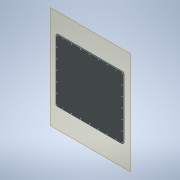
# Autodesk Inventor part: Крышка картера 2
Saved by Autodesk Inventor 2021 (Build 250183000, 183)
## iProperties
Created: 2020-12-12
Part Number: Крышка картера 2
Material: Чугун, серый
Document SubType Name: Modeling
Designer: Тимоха
Mass: 32984 g
Surface Area: 9566.62 cm^2
Volume: 4613.15 cm^3
Density: 7.15 g/cm^3
Appearance: Чугун серый
Author: Тимоха
Autodesk Inventor part; units mm, degrees
ref_plane "YZ Plane" through (0, 0, 0) normal (1, 0, 0) x (0, 1, 0)
ref_plane "XZ Plane" through (0, 0, 0) normal (0, 1, 0) x (-1, 0, 0)
ref_plane "XY Plane" through (0, 0, 0) normal (0, 0, 1) x (1, 0, 0)
ref_plane "РабПлоскость1" through (0, 0, 0) normal (0, 0, 1) x (1, 0, 0)
sketch "Эскиз1" plane through (0, 0, 0) normal (0, 0, 1) x (1, 0, 0)
  circle A0 centre (340, 472) radius 4 projected
  circle A1 centre (340, 367) radius 4 projected
  circle A2 centre (340, 322.8) radius 4 projected
  circle A3 centre (340, 218.5) radius 4 projected
  circle A4 centre (340, 114.2) radius 4 projected
  circle A5 centre (340, 9.9) radius 4 projected
  circle A6 centre (340, -94.4) radius 4 projected
  circle A7 centre (340, -198.7) radius 4 projected
  circle A8 centre (340, -303) radius 4 projected
  circle A9 centre (340, -347) radius 4 projected
  circle A10 centre (340, -407) radius 4 projected
  circle A11 centre (340, -467) radius 4 projected
  circle A12 centre (278, 472) radius 4 projected
  circle A13 centre (185, 472) radius 4 projected
  circle A14 centre (92, 472) radius 4 projected
  circle A15 centre (-1, 472) radius 4 projected
  circle A16 centre (-94, 472) radius 4 projected
  circle A17 centre (-187, 472) radius 4 projected
  circle A18 centre (-280, 472) radius 4 projected
  circle A19 centre (-340, 472) radius 4 projected
  circle A20 centre (-340, 367) radius 4 projected
  circle A21 centre (-340, 322.8) radius 4 projected
  circle A22 centre (-340, 218.5) radius 4 projected
  circle A23 centre (-340, 114.2) radius 4 projected
  circle A24 centre (-340, 9.9) radius 4 projected
  circle A25 centre (-340, -94.4) radius 4 projected
  circle A26 centre (-340, -198.7) radius 4 projected
  circle A27 centre (-340, -303) radius 4 projected
  circle A28 centre (-340, -347) radius 4 projected
  circle A29 centre (-340, -407) radius 4 projected
  circle A30 centre (-340, -467) radius 4 projected
  line L0 (165, -460) -> (165, -485) projected
  line L1 (185, -485) -> (165, -485) projected
  line L2 (185, -475) -> (185, -485) projected
  line L3 (185, -475) -> (380, -475) projected
  line L4 (380, -475) -> (380, 475) projected
  line L5 (380, 475) -> (350, 475) projected
  line L6 (350, 475) -> (350, 485) projected
  line L7 (-350, 485) -> (350, 485) projected
  line L8 (-350, 475) -> (-350, 485) projected
  line L9 (-350, 475) -> (-380, 475) projected
  line L10 (-380, 475) -> (-380, -475) projected
  line L11 (-380, -475) -> (-185, -475) projected
  line L12 (-185, -475) -> (-185, -485) projected
  line L13 (-165, -485) -> (-185, -485) projected
  line L14 (-165, -485) -> (-165, -460) projected
  line L15 (-165, -460) -> (-330, -460) projected
  line L16 (-330, 460) -> (-330, -460) projected
  line L17 (-330, 460) -> (330, 460) projected
  line L18 (330, -460) -> (330, 460) projected
  line L19 (330, -460) -> (165, -460) projected
  circle A31 centre (278, -303) radius 4 projected
  circle A32 centre (185, -303) radius 4 projected
  circle A33 centre (92, -303) radius 4 projected
  circle A34 centre (-1, -303) radius 4 projected
  circle A35 centre (-94, -303) radius 4 projected
  circle A36 centre (-187, -303) radius 4 projected
  circle A37 centre (-280, -303) radius 4 projected
  circle A38 centre (278, -347) radius 4 projected
  circle A39 centre (185, -347) radius 4 projected
  circle A40 centre (92, -347) radius 4 projected
  circle A41 centre (-1, -347) radius 4 projected
  circle A42 centre (-94, -347) radius 4 projected
  circle A43 centre (-187, -347) radius 4 projected
  circle A44 centre (-280, -347) radius 4 projected
  line L20 (-330, -291) -> (-330, -359) projected
  line L21 (-330, -359) -> (330, -359) projected
  line L22 (330, -291) -> (330, -359) projected
  line L23 (-330, -291) -> (330, -291) projected
  circle A45 centre (278, 367) radius 4 projected
  circle A46 centre (185, 367) radius 4 projected
  circle A47 centre (92, 367) radius 4 projected
  circle A48 centre (-1, 367) radius 4 projected
  circle A49 centre (-94, 367) radius 4 projected
  circle A50 centre (-187, 367) radius 4 projected
  circle A51 centre (-280, 367) radius 4 projected
  circle A52 centre (278, 323) radius 4 projected
  circle A53 centre (185, 323) radius 4 projected
  circle A54 centre (92, 323) radius 4 projected
  circle A55 centre (-1, 323) radius 4 projected
  circle A56 centre (-94, 323) radius 4 projected
  circle A57 centre (-187, 323) radius 4 projected
  circle A58 centre (-280, 323) radius 4 projected
  line L24 (-330, 379) -> (-330, 311) projected
  line L25 (-330, 311) -> (330, 311) projected
  line L26 (330, 379) -> (330, 311) projected
  line L27 (-330, 379) -> (330, 379) projected
  circle A59 centre (-340, 322.8) radius 14
  circle A60 centre (-340, -303) radius 14
  circle A61 centre (340, -303) radius 14
  circle A62 centre (340, 322.8) radius 14
  line L28 (340, 336.8) -> (-340, 336.8)
  line L29 (-354, 322.8) -> (-354, -303)
  line L30 (-340, -317) -> (340, -317)
  line L31 (354, -303) -> (354, 322.8)
  point P0 (0, 0)
  dimension "d0" = 10
  dimension "d1" = 10
  dimension "d2" = 10
  dimension "d3" = 10
  constraints: 8 end point, 8 point on circle, 5 tangent, 4 centre point
  measures "d0" radial gap between concentric circles of A21 A59
  measures "d1" radial gap between concentric circles of A27 A60
  measures "d2" radial gap between concentric circles of A8 A61
  measures "d3" radial gap between concentric circles of A2 A62
extrude "Выдавливание1" add sketch "Эскиз1" along normal blind 10 contours L30 L16 A60 L23 L18 A61 | L18 A61 L30 | A61 L18 | L18 A61 | L30 A60 L16 | L18 A62 L31 A61 | A60 L16 | L16 A60 | L23 L16 L25 L18 | A60 L29 A59 L16 | A62 L18 | L25 L16 A59 L28 L18 A62 | A59 L16 | A62 L18 L28 | A62 L18 | L28 L16 A59 | L16 A59
